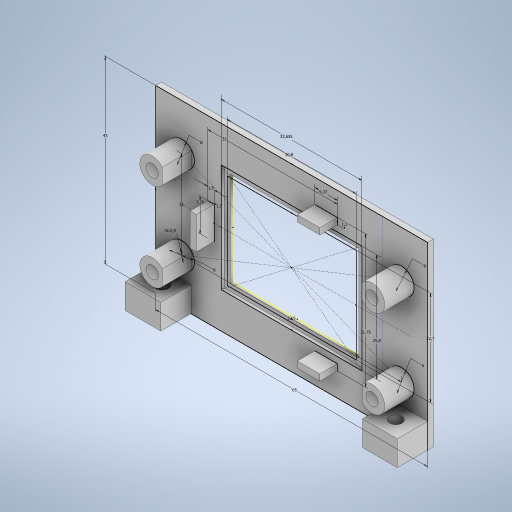
# Autodesk Inventor part: clamp
Saved by Autodesk Inventor 2024 (Build 280153000, 153)
## iProperties
Created: 2024-09-23
Part Number: clamp
Material: Generic
Document SubType Name: Modeling
Designer: PC
Density: 1 g/cm^3
Appearance: Default
Author: PC
Autodesk Inventor part; units mm, degrees
ref_plane "YZ Plane" through (0, 0, 0) normal (1, 0, 0) x (0, 1, 0)
ref_plane "XZ Plane" through (0, 0, 0) normal (0, 1, 0) x (-1, 0, 0)
ref_plane "XY Plane" through (0, 0, 0) normal (0, 0, 1) x (1, 0, 0)
sketch "Sketch1" plane through (0, 0, 0) normal (0, 0, 1) x (1, 0, 0)
  circle A0 centre (0, 0) radius 1.45
  line L0 (0, 0) -> (29.0858, 0) construction
  line L1 (0, 0) -> (0, 12.0151) construction
  circle A1 centre (52.5, 0) radius 1.45
  circle A2 centre (0, 21) radius 1.45
  circle A3 centre (52.5, 21) radius 1.45
  line L2 (9.4225, 23.4) -> (43.0775, 23.4)
  line L3 (43.0775, 23.4) -> (43.0775, -2.4)
  line L4 (43.0775, -2.4) -> (9.4225, -2.4)
  line L5 (9.4225, -2.4) -> (9.4225, 23.4)
  line L6 (0, 0) -> (52.5, 0) construction
  line L7 (0, 0) -> (0, 21) construction
  line L8 (31.8525, 26.375) -> (37.2225, 26.375)
  line L9 (37.2225, 26.375) -> (37.2225, 24.875)
  line L10 (37.2225, 24.875) -> (31.8525, 24.875)
  line L11 (31.8525, 24.875) -> (31.8525, 26.375)
  line L12 (0, 10.5) -> (54.8586, 10.5) construction
  line L13 (31.8525, -5.375) -> (37.2225, -5.375)
  line L14 (37.2225, -5.375) -> (37.2225, -3.875)
  line L15 (37.2225, -3.875) -> (31.8525, -3.875)
  line L16 (31.8525, -3.875) -> (31.8525, -5.375)
  line L17 (6.2225, 14.375) -> (7.7225, 14.375)
  line L18 (7.7225, 14.375) -> (7.7225, 6.625)
  line L19 (7.7225, 6.625) -> (6.2225, 6.625)
  line L20 (6.2225, 6.625) -> (6.2225, 14.375)
  line L21 (-6.25, 32) -> (58.75, 32)
  line L22 (58.75, 32) -> (58.75, -11)
  line L23 (58.75, -11) -> (-6.25, -11)
  line L24 (-6.25, -11) -> (-6.25, 32)
  line L25 (10.85, 21.85) -> (41.65, 21.85)
  line L26 (41.65, 21.85) -> (41.65, -0.85)
  line L27 (41.65, -0.85) -> (10.85, -0.85)
  line L28 (10.85, -0.85) -> (10.85, 21.85)
  line L29 (9.4225, -2.4) -> (43.0775, 23.4) construction
  line L30 (9.4225, 23.4) -> (43.0775, -2.4) construction
  circle A4 centre (0, 0) radius 3
  circle A5 centre (0, 21) radius 3
  circle A6 centre (52.5, 21) radius 3
  circle A7 centre (52.5, 0) radius 3
  line L31 (0, 0) -> (52.5, 21) construction
  line L32 (0, 21) -> (52.5, 0) construction
  point P0 (9.4225, 10.5)
  point P1 (26.25, 0)
  point P2 (26.25, -2.4)
  point P3 (7.7225, 10.5)
  point P4 (37.2225, 25.625)
  point P5 (26.25, 10.5)
  point P6 (26.25, 21.85)
  point P7 (26.25, 10.5)
  point P8 (41.65, 10.5)
  point P9 (-6.25, 10.5)
  point P10 (26.25, 32)
  dimension "d0" = 2.9
  dimension "d3" = 52.5
  dimension "d6" = 21
  dimension "d9" = 33.655
  dimension "d10" = 25.8
  dimension "d11" = 5.37
  dimension "d12" = 1.5
  dimension "d15" = 7.75
  dimension "d16" = 31.75
  dimension "d17" = 31
  dimension "d18" = 1.5
  dimension "d19" = 1.7
  dimension "d20" = 30.8
  dimension "d21" = 22.7
  dimension "d22" = 43
  dimension "d23" = 65
  dimension "d31" = 6
  dimension "d32" = 6
  dimension "d33" = 6
  dimension "d34" = 6
  constraints: 66 end point, 12 midpoint, 10 parallel, 9 horizontal, 8 centre point, 5 coincident, 5 perpendicular, 4 symmetric about line, 3 horizontal alignment, 3 vertical, 3 vertical alignment, 1 point on line, 6 other
  measures "d0" diameter of A0
  measures "d3" distance of L0.start L6.end
  measures "d6" distance of L0.start L7.end
  measures "d9" distance of L2.start L2.end
  measures "d10" distance of L2.end L3.end
  measures "d11" distance of L8.start L8.end
  measures "d12" distance of L8.end L9.end
  measures "d15" distance of L19.end L17.start
  measures "d16" distance between parallel lines of L13 L8
  measures "d17" distance from line of L20 point (37.223, 25.625)
  measures "d18" distance of L17.start L17.end
  measures "d19" distance between parallel lines of L5 L18
  measures "d20" distance of L25.start L25.end
  measures "d21" distance of L25.end L26.end
  measures "d22" distance of L23.end L21.start
  measures "d23" distance between parallel lines of L22 L24
  measures "d31" diameter of A4
  measures "d32" diameter of A5
  measures "d33" diameter of A6
  measures "d34" diameter of A7
extrude "Extrusion1" add sketch "Sketch1" against normal blind 1.4 contours L8 L9 L10 L11 | L16 L15 L14 L13 | L17 L18 L19 L20 | L21 L22 L23 L24 | A4 | A5 | A6 | A7
extrude "Extrusion2" add sketch "Sketch1" along normal blind 4.2 contours L8 L9 L10 L11 | L16 L15 L14 L13 | L17 L18 L19 L20
extrude "Extrusion3" add sketch "Sketch1" along normal blind 7 contours A4 | A5 | A6 | A7
sketch "Sketch3" plane through (0, 21, 7) normal (0, 0, 1) x (1, 0, 0)
  line L0 (2.35, 3.2266) -> (50.15, 3.2266)
  line L1 (50.15, 3.2266) -> (50.15, -23.7734)
  line L2 (50.15, -23.7734) -> (2.35, -23.7734)
  line L3 (2.35, -23.7734) -> (2.35, 3.2266)
  circle A0 centre (0, 0) radius 3 projected
  circle A1 centre (52.5, 0) radius 3 projected
  line L4 (2.35, -23.7734) -> (50.15, 3.2266) construction
  line L5 (2.35, 3.2266) -> (50.15, -23.7734) construction
  line L6 (9.4225, 2.4) -> (43.0775, 2.4) construction
  line L7 (4.5388, -3.9941) -> (9.4225, -3.9941)
  line L8 (9.4225, -3.9941) -> (9.4225, -17.6824)
  line L9 (9.4225, -17.6824) -> (4.5388, -17.6824)
  line L10 (4.5388, -17.6824) -> (4.5388, -3.9941)
  point P0 (0, -21)
  point P1 (26.25, -10.2734)
  point P2 (26.25, 2.4)
  point P3 (2.35, 1.8648)
  point P4 (2.35, -1.8648)
  point P5 (50.15, -1.8648)
  point P6 (50.15, 1.8648)
  dimension "d37" = 47.8
  dimension "d40" = 27
  constraints: 20 end point, 4 parallel, 2 horizontal, 2 midpoint, 2 perpendicular, 1 vertical alignment
  measures "d37" distance of L0.start L0.end
  measures "d40" distance between parallel lines of L2 L0
extrude "Extrusion4" cut sketch "Sketch3" against normal up to surface (7 mm away) contours L0 L1 A1 L2 L3 A0 | A0 L3 | L1 A1 picked at (2.4683, -0.4324) picked at (50.0317, -0.4324)
extrude "Extrusion5" add sketch "Sketch1" against normal blind 1.4 contours L2 L3 L4 L5
extrude "Extrusion6" cut sketch "Sketch1" against normal blind 0.7 contours L2 L3 L4 L5
sketch "Sketch5" plane through (0, 0, 0) normal (0, 0, 1) x (1, 0, 0)
  line L0 (58.75, -11) -> (-6.25, -11) construction
  line L1 (48.0157, -11) -> (48.0157, 32) construction
  line L2 (-6.25, 32) -> (58.75, 32) construction
  point P0 (0, 0)
  constraints: 2 end point, 2 point on line, 1 vertical
sketch "Sketch2" plane through (-6.25, -11, 0) normal (0, -1, 0) x (1, 0, 0)
  circle A0 centre (60.9, 3.5) radius 1.45
  circle A1 centre (5.1, 3.5) radius 1.5013
  line L0 (0, 0) -> (65, 0) projected
  line L1 (5.1, 3.5) -> (60.9, 3.5) construction
  line L2 (65, 0) -> (56.7123, 0)
  line L3 (56.7123, 0) -> (56.7123, 7.2261)
  line L4 (56.7123, 7.2261) -> (65, 7.2261)
  line L5 (65, 7.2261) -> (65, 0)
  line L6 (8.4882, 7.2261) -> (0, 7.2261)
  line L7 (0, 7.2261) -> (0, 0)
  line L8 (0, 0) -> (8.4882, 0)
  line L9 (8.4882, 0) -> (8.4882, 7.2261)
  point P0 (6.25, 0)
  point P1 (56.4, 7)
  dimension "d28" = 2.9
  dimension "d29" = 55.8
  dimension "d30" = 3.5
  dimension "d47" = 4.5
  constraints: 18 end point, 4 parallel, 3 horizontal, 2 centre point, 2 perpendicular, 1 point on line
  measures "d28" diameter of A0
  measures "d29" distance of L1.end L1.start
  measures "d30" distance from line of L0 L1.start
  measures "d47" horizontal distance of L1.end point (56.4, 7)
sketch "Sketch4" plane through (0, 0, -1.4) normal (0, 0, -1) x (-1, 0, 0)
  line L0 (-7.2429, 23.3728) -> (-45.2571, 23.3728)
  line L1 (-45.2571, 23.3728) -> (-45.2571, -2.3728)
  line L2 (-45.2571, -2.3728) -> (-7.2429, -2.3728)
  line L3 (-7.2429, -2.3728) -> (-7.2429, 23.3728)
  line L4 (-2.9215, 28.8809) -> (-49.5785, 28.8809)
  line L5 (-49.5785, 28.8809) -> (-49.5785, -7.8809)
  line L6 (-49.5785, -7.8809) -> (-2.9215, -7.8809)
  line L7 (-2.9215, -7.8809) -> (-2.9215, 28.8809)
  line L8 (-10.85, -0.85) -> (-41.65, -0.85) projected
  line L9 (-10.85, 21.85) -> (-10.85, -0.85) projected
  point P0 (0, 0)
  point P1 (-26.25, -2.3728)
  point P2 (-26.25, -0.85)
  point P3 (-10.85, 10.5)
  point P4 (-7.2429, 10.5)
  point P5 (-2.9215, 10.5)
  point P6 (-26.25, -7.8809)
  point P7 (-26.25, -0.85)
  constraints: 16 end point, 7 midpoint, 4 parallel, 3 vertical alignment, 2 horizontal, 2 horizontal alignment, 2 perpendicular
extrude "Extrusion7" add sketch "Sketch2" against normal blind 6
equation "\"d0\" = m3"
equation "\"d28\" = m3"
equation "\"m3\" = 2.9"
body "Solid1"
